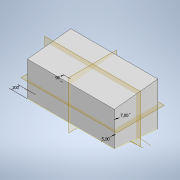
# Autodesk Inventor part: Telaio
Saved by Autodesk Inventor 2021 (Build 250183000, 183)
## iProperties
Created: 2021-05-04
Part Number: Telaio
Material: Generic
Document SubType Name: Modeling
Designer: andre
Density: 1 g/cm^3
Appearance: Default
Author: andre
Autodesk Inventor part; units mm, degrees
sketch "Sketch5" plane through (0, 0, 0) normal (0, 0, 1) x (1, 0, 0)
  line L0 (-500, -250) -> (500, -250)
  line L1 (500, -250) -> (500, 250)
  line L2 (500, 250) -> (-500, 250)
  line L3 (-500, 250) -> (-500, -250)
  line L4 (-500, -250) -> (500, 250) construction
  line L5 (500, -250) -> (-500, 250) construction
  point P0 (0, 0)
  dimension "d11" = 1000
  dimension "d12" = 500
  constraints: 12 end point, 2 midpoint, 2 parallel, 1 horizontal, 1 perpendicular
  measures "d11" distance of L1.end L2.end
  measures "d12" distance of L0.end L1.end
extrude "Extrusion3" add sketch "Sketch5" along normal mid plane 500
sketch "Sketch6" plane through (500, -250, 250) normal (1, 0, 0) x (0, 0, -1)
  line L0 (0, 0) -> (0, 500) construction
  line L1 (500, 0) -> (500, 500) construction
  line L2 (0, 52.5521) -> (500, 0)
  line L3 (500, 0) -> (0, 0)
  line L4 (0, 0) -> (0, 52.5521)
  point P0 (250, 250)
  dimension "d15" = 6
  constraints: 6 end point, 1 horizontal, 1 perpendicular, 1 point on line
  measures "d15" angle of L3 L2
extrude "Extrusion4" cut sketch "Sketch6" against normal up to next
mirror "Mirror2" about plane through (0, 0, 0) normal (0, 1, 0) of "Extrusion4"
sketch "Sketch7" plane through (-500, -250, -250) normal (0, -0.9945, 0.1045) x (1, 0, 0)
  line L0 (0, 402.7541) -> (1000, 315.2655)
  line L1 (1000, 502.7541) -> (1000, 0) construction
  line L2 (0, 502.7541) -> (1000, 502.7541) construction
  line L3 (0, 0) -> (0, 502.7541) construction
  point P0 (500, 274.7626)
  dimension "d18" = 5
  dimension "d19" = 100
  constraints: 2 end point, 2 point on line
  measures "d18" angle of L2 L0
  measures "d19" distance from line of L2 L0.start
sketch "Sketch8" plane through (-500, -250, -250) normal (0, -0.9945, 0.1045) x (1, 0, 0)
  line L0 (0, 0) -> (0, 502.7541) construction
  line L1 (0, 90) -> (1000, 212.7846)
  line L2 (1000, 502.7541) -> (1000, 0) construction
  line L3 (1000, 0) -> (0, 0) construction
  point P0 (500, 274.7626)
  dimension "d20" = 7
  dimension "d21" = 90
  constraints: 2 end point, 2 point on line
  measures "d20" angle of L3 L1
  measures "d21" distance from line of L1.start L3
body "Solid2"
